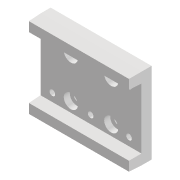
# Autodesk Inventor part: 20_Cube_Insert_Linear_Stage_NEMA11_china_xymount
Saved by Autodesk Inventor 2022 (Build 260153000, 153)
## iProperties
Created: 2022-01-15
Part Number: 20_Cube_Insert_Linear_Stage_NEMA11_china_xymount
Material: Generisch
Document SubType Name: Modeling
Designer: diederichbenedict
Density: 1 g/cm^3
Appearance: Vorgabe
Author: diederichbenedict
Autodesk Inventor part; units mm, degrees
ref_plane "YZ Plane" through (0, 0, 0) normal (1, 0, 0) x (0, 1, 0)
ref_plane "XZ Plane" through (0, 0, 0) normal (0, 1, 0) x (-1, 0, 0)
ref_plane "Arbeitsebene1" through (0, 0, 0) normal (0, 0, 1) x (1, 0, 0)
sketch "Skizze1" plane through (0, 0, 0) normal (0, 0, 1) x (1, 0, 0)
  line L0 (15, 26.0506) -> (15, 58.2506) projected
  line L1 (15, 58.2506) -> (-15, 58.2506) projected
  line L2 (-15, 58.2506) -> (-15, 26.0506) projected
  line L3 (-15, 26.0506) -> (15, 26.0506) projected
  circle A0 centre (10, 32.1506) radius 1.25 construction
  circle A1 centre (-10, 32.1506) radius 1.25 construction
  circle A2 centre (-10, 52.1506) radius 1.25 construction
  circle A3 centre (10, 52.1506) radius 1.25 construction
  circle A4 centre (7.5, 38.0506) radius 3.25 construction
  circle A5 centre (7.5, 46.2506) radius 3.25 construction
  circle A6 centre (-7.5, 38.0506) radius 3.25 construction
  circle A7 centre (-7.5, 46.2506) radius 3.25 construction
  line L4 (-65, 27.1506) -> (-65, 57.1506) projected
  circle A8 centre (10, 32.1506) radius 1.25
  circle A9 centre (-10, 32.1506) radius 1.25
  circle A10 centre (-10, 52.1506) radius 1.25
  circle A11 centre (10, 52.1506) radius 1.25
  line L5 (15, 58.2506) -> (25, 58.2506)
  line L6 (25, 58.2506) -> (25, 26.0506)
  line L7 (25, 26.0506) -> (15, 26.0506)
  line L8 (15, 26.0506) -> (15, 58.2506)
  line L9 (-15, 58.2506) -> (-25, 58.2506)
  line L10 (-25, 58.2506) -> (-25, 26.0506)
  line L11 (-25, 26.0506) -> (-15, 26.0506)
  line L12 (-15, 26.0506) -> (-15, 58.2506)
  line L13 (25, 26.0506) -> (-25, 26.0506)
  line L14 (-25, 26.0506) -> (-25, 22.0506)
  line L15 (-25, 22.0506) -> (25, 22.0506)
  line L16 (25, 22.0506) -> (25, 26.0506)
  line L17 (25, 58.2506) -> (-25, 58.2506)
  line L18 (-25, 58.2506) -> (-25, 62.2506)
  line L19 (-25, 62.2506) -> (25, 62.2506)
  line L20 (25, 62.2506) -> (25, 58.2506)
  point P0 (0, 0)
  dimension "d19" = 10
  dimension "d20" = 10
  dimension "d26" = 4
  dimension "d27" = 4
  constraints: 32 end point, 8 parallel, 4 centre point, 4 coincident, 4 concentric, 4 horizontal, 4 perpendicular, 1 point on line
  measures "d19" distance of L6.end L7.end
  measures "d20" distance of L11.end L10.end
  measures "d26" distance of L10.end L14.end
  measures "d27" distance of L17.end L18.end
ref_plane "Arbeitsebene2" through (-72, 28.2506, 5) normal (0, 0, -1) x (0, 1, 0)
extrude "Extrusion1" add sketch "Skizze1" along normal up to surface (5 mm away)
sketch "Skizze2" plane through (-15, 58.2506, 5) normal (0, 0, 1) x (1, 0, 0)
  circle A0 centre (25, -26.1) radius 1.25 projected
  circle A1 centre (5, -26.1) radius 1.25 projected
  circle A2 centre (5, -6.1) radius 1.25 projected
  circle A3 centre (25, -6.1) radius 1.25 projected
  point P0 (15, -58.2506)
hole "Bohrung1" at (10, 32.1506, 5) at (-10, 32.1506, 5) at (-10, 52.1506, 5) at (10, 52.1506, 5) direction (0, 0, -1) diameter 2.8 end through all counterbore diameter 7 counterbore depth 3
sketch "Skizze3" plane through (-15, 58.2506, 5) normal (0, 0, 1) x (1, 0, 0)
  circle A0 centre (14.8208, -23.6) radius 1.7 projected
  circle A1 centre (14.8208, -8.6) radius 1.7 projected
  circle A2 centre (5, -6.1) radius 3.5 projected
  circle A3 centre (25, -26.1) radius 3.5 projected
  circle A4 centre (5, -26.1) radius 3.5 projected
  circle A5 centre (25, -6.1) radius 3.5 projected
  line L0 (-10, 0) -> (-10, -32.2) projected
  line L1 (-10, -16.1) -> (40, -16.1)
  line L2 (40, -32.2) -> (40, 0) projected
  circle A6 centre (14.8208, -5.1) radius 1.5853
  circle A7 centre (14.8208, -27.1) radius 2.0333
  point P0 (15, -58.2506)
  dimension "d24" = 11
  dimension "d25" = 11
  constraints: 2 centre point, 2 end point, 2 midpoint
  measures "d24" distance from line of A7.centre L1
  measures "d25" distance from line of A6.centre L1
hole "Bohrung2" at (-0.1792, 31.1506, 5) at (-0.1792, 53.1506, 5) direction (0, 0, -1) diameter 2.8 end through all
pattern_linear "Rechteckige Anordnung1" count 3 spacing 19 along (-1, 0, 0) of "Bohrung2" first direction both ways yes
sketch "Skizze5" plane through (-25, 62.2506, 5) normal (0, 0, 1) x (1, 0, 0)
  line L0 (-41, -5.1) -> (47, -5.1) projected
  line L1 (-24.541, -42.8) -> (44.8306, -42.8) projected
  line L2 (16.25, -40.0792) -> (10.75, -40.0792) projected
  line L3 (0, -40.2) -> (50, -40.2) projected
  line L4 (50, 0) -> (0, 0) projected
  line L5 (-41, -35.1) -> (47, -35.1) projected
  line L6 (50, 0) -> (0, 0)
  line L7 (0, 0) -> (0, -5.1)
  line L8 (0, -5.1) -> (50, -5.1)
  line L9 (50, -5.1) -> (50, 0)
  line L10 (0, -40.2) -> (50, -40.2) projected
  line L11 (0, 0) -> (0, -40.2) projected
  line L12 (50, -40.2) -> (0, -40.2)
  line L13 (0, -40.2) -> (0, -35.1)
  line L14 (0, -35.1) -> (50, -35.1)
  line L15 (50, -35.1) -> (50, -40.2)
  point P0 (25, -62.2506)
  point P1 (47, -5.1)
  constraints: 16 end point, 4 parallel, 4 point on line, 2 horizontal, 2 perpendicular
extrude "Extrusion3" add sketch "Skizze5" along normal blind 6 draft -2
sketch "Skizze6" plane through (0, 0, 0) normal (0, 0, -1) x (-1, 0, 0)
  circle A0 centre (19.1792, 31.1506) radius 1.4 projected
  circle A1 centre (19.1792, 53.1506) radius 1.4 projected
  circle A2 centre (-18.8208, 31.1506) radius 1.4 projected
  circle A3 centre (-18.8208, 53.1506) radius 1.4 projected
  circle A4 centre (0.1792, 31.1506) radius 1.4 projected
  circle A5 centre (0.1792, 53.1506) radius 1.4 projected
  circle A6 centre (10, 52.1506) radius 1.4 projected
  circle A7 centre (-10, 32.1506) radius 1.4 projected
  circle A8 centre (10, 32.1506) radius 1.4 projected
  circle A9 centre (-10, 52.1506) radius 1.4 projected
  line L0 (25, 62.2506) -> (25, 22.0506) projected
  line L1 (-25, 62.2506) -> (25, 62.2506) projected
  line L2 (-25, 22.0506) -> (-25, 62.2506) projected
  line L3 (25, 22.0506) -> (-25, 22.0506) projected
  point P0 (0, 0)
extrude "Extrusion4" add sketch "Skizze6" along normal blind 2
